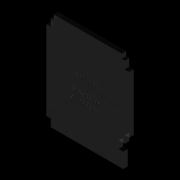
# Autodesk Inventor part: SideFaceBottomNM
Saved by Autodesk Inventor 2019 (Build 230136000, 136)
## iProperties
Created: 2019-05-08
Part Number: SideFaceBottomNM
Material: Acrylic, Clear
Document SubType Name: Modeling
Designer: super pig
Density: 1.19 g/cm^3
Appearance: Transparent - Black
Mass: 11.9621 g
Surface Area: 75.9473 cm^2
Volume: 10.0522 cm^3
Name: Bottom Face Cover
Author: super pig
Autodesk Inventor part; units mm, degrees
note: some values were not read from the file. Chosen so that the rebuilt part matches the saved one: direction of "Emboss1"; direction of "Emboss2".
ref_plane "YZ Plane" through (0, 0, 0) normal (1, 0, 0) x (0, 1, 0)
ref_plane "XZ Plane" through (0, 0, 0) normal (0, 1, 0) x (-1, 0, 0)
ref_plane "XY Plane" through (0, 0, 0) normal (0, 0, 1) x (1, 0, 0)
sketch "Sketch1" plane through (0, 0, 0) normal (0, 0, 1) x (1, 0, 0)
  line L0 (45, -52.75) -> (48, -52.75) projected
  line L1 (45, -52.75) -> (45, -62.75) projected
  line L2 (45, -62.75) -> (48, -62.75) projected
  line L3 (48, -52.75) -> (48, -62.75) projected
  line L4 (45, -47.75) -> (45, -52.75) projected
  line L5 (45, -52.75) -> (48, -52.75) projected
  line L6 (48, -47.75) -> (48, -52.75) projected
  line L7 (45, -47.75) -> (48, -47.75) projected
  line L8 (49, -42.75) -> (49, -47.75) projected
  line L9 (52, -42.75) -> (52, -47.75) projected
  line L10 (49, -42.75) -> (52, -42.75) projected
  line L11 (49, -5) -> (52, -5) projected
  line L12 (49, -5) -> (49, -42.75) projected
  line L13 (49, -42.75) -> (52, -42.75) projected
  line L14 (52, -5) -> (52, -42.75) projected
  line L15 (49, 0) -> (49, -5) projected
  line L16 (49, -5) -> (52, -5) projected
  line L17 (52, 0) -> (52, -5) projected
  line L18 (49, 0) -> (52, 0) projected
  line L19 (2, 3) -> (47, 3)
  line L20 (2, 0) -> (47, 0)
  line L21 (0, -5) -> (0, 0) projected
  line L22 (0, 0) -> (-3, 0) projected
  line L23 (-3, -5) -> (-3, 0) projected
  line L24 (0, -5) -> (-3, -5) projected
  line L25 (0, -57.75) -> (-3, -57.75) projected
  line L26 (0, -57.75) -> (0, -5) projected
  line L27 (-3, -57.75) -> (-3, -5) projected
  line L28 (0, -62.75) -> (0, -57.75) projected
  line L29 (0, -57.75) -> (-3, -57.75) projected
  line L30 (-3, -62.75) -> (-3, -57.75) projected
  line L31 (0, -62.75) -> (-3, -62.75) projected
  line L32 (48, -47.75) -> (49, -47.75)
  line L33 (45, -62.75) -> (0, -62.75)
  line L34 (49, -47.75) -> (52, -47.75) projected
  line L35 (0, -5) -> (-3, -5) projected
  line L36 (47, 3) -> (52, 3) projected
  line L37 (47, 0) -> (47, 3) projected
  line L38 (47, 0) -> (52, 0) projected
  line L39 (52, 0) -> (52, 3) projected
  line L40 (-3, 0) -> (2, 0) projected
  line L41 (2, 0) -> (2, 3) projected
  line L42 (-3, 3) -> (2, 3) projected
  line L43 (-3, 0) -> (-3, 3) projected
  constraints: 8 end point, 1 collinear, 1 horizontal
extrude "Extrusion1" add sketch "Sketch1" along normal blind 3 contours L0 L3 L2 L1 | L1 L33 L28 L26 L21 L40 L20 L38 L15 L12 L8 L32 L7 L4 | L25 L27 L24 L26 | L12 L11 L14 L10 | L41 L19 L37 L20
sketch "Sketch2" plane through (0, 0, 3) normal (0, 0, 1) x (1, 0, 0)
  circle A0 centre (38, -35.75) radius 4
  circle A1 centre (38, -23.75) radius 4
  line L0 (49, -47.75) -> (49, -42.75) projected
  line L1 (49, -42.75) -> (52, -42.75) projected
  point P0 (0, 0)
  point P1 (49, -5)
  dimension "d3" = 8
  dimension "d4" = 12
  dimension "d5" = 7
  dimension "d13" = 11
  constraints: 2 centre point, 1 equal radius, 1 vertical alignment
  measures "d3" diameter of A0
  measures "d4" distance of A0.centre A1.centre
  measures "d5" distance from line of L1 A0.centre
  measures "d13" distance from line of A0.centre L0
extrude "Extrusion2" cut sketch "Sketch2" against normal through all
sketch "Sketch3" plane through (0, 0, 3) normal (0, 0, 1) x (1, 0, 0)
  line L0 (45, -62.25) -> (0, -62.25) construction
  line L1 (0, -62.25) -> (0, -49.7711) construction
  line L2 (0, -49.7711) -> (45, -49.7711) construction
  line L3 (45, -49.7711) -> (45, -62.25) construction
  line L4 (45, -52.75) -> (45, -47.75) construction
  line L5 (0, -57.75) -> (0, -62.75) construction
  line L6 (0, -62.75) -> (48, -62.75) construction
  line L7 (42.4636, -61.6943) -> (42.9177, -61.6943)
  line L8 (42.9177, -61.6943) -> (42.9177, -60.9405)
  line L9 (42.9177, -60.9405) -> (43.1386, -60.9405)
  line L10 (43.1386, -60.9405) -> (43.1386, -61.6943)
  line L11 (43.1386, -61.6943) -> (43.5926, -61.6943)
  line L12 (43.5926, -61.6943) -> (43.5926, -61.7539)
  line L13 (43.5926, -61.7539) -> (43.0702, -62.3359)
  line L14 (43.0702, -62.3359) -> (42.9983, -62.3359)
  line L15 (42.9983, -62.3359) -> (42.4636, -61.7521)
  line L16 (42.4636, -61.7521) -> (42.4636, -61.6943)
  line L17 (38.7379, -59.294) -> (39.6954, -59.294)
  line L18 (39.6954, -59.294) -> (39.6954, -59.541)
  line L19 (39.6954, -59.541) -> (39.3488, -59.541)
  line L20 (39.3488, -59.541) -> (39.3488, -61.3891)
  line L21 (39.3488, -61.3891) -> (39.6954, -61.3891)
  line L22 (39.6954, -61.3891) -> (39.6954, -61.638)
  line L23 (39.6954, -61.638) -> (38.7379, -61.638)
  line L24 (38.7379, -61.638) -> (38.7379, -61.3891)
  line L25 (38.7379, -61.3891) -> (39.0845, -61.3891)
  line L26 (39.0845, -61.3891) -> (39.0845, -59.541)
  line L27 (39.0845, -59.541) -> (38.7379, -59.541)
  line L28 (38.7379, -59.541) -> (38.7379, -59.294)
  line L29 (36.48, -59.315) -> (36.6983, -59.315)
  line L30 (36.6983, -59.315) -> (37.9661, -61.1746)
  line L31 (37.9661, -61.1746) -> (37.9661, -59.315)
  line L32 (37.9661, -59.315) -> (38.2304, -59.315)
  line L33 (38.2304, -59.315) -> (38.2304, -61.6112)
  line L34 (38.2304, -61.6112) -> (38.0121, -61.617)
  line L35 (38.0121, -61.617) -> (36.7443, -59.7574)
  line L36 (36.7443, -59.7574) -> (36.7443, -61.615)
  line L37 (36.7443, -61.615) -> (36.48, -61.615)
  line L38 (36.48, -61.615) -> (36.48, -59.315)
  line L39 (34.2068, -59.7651) -> (34.699, -59.294)
  line L40 (34.699, -59.294) -> (35.5474, -59.294)
  line L41 (35.5474, -59.294) -> (36.0223, -59.7498)
  line L42 (36.0223, -59.7498) -> (35.848, -59.9145)
  line L43 (35.848, -59.9145) -> (35.442, -59.541)
  line L44 (35.442, -59.541) -> (34.8043, -59.541)
  line L45 (34.8043, -59.541) -> (34.5515, -59.7651)
  line L46 (34.5515, -59.7651) -> (36.0376, -61.1631)
  line L47 (36.0376, -61.1631) -> (35.5474, -61.638)
  line L48 (35.5474, -61.638) -> (34.699, -61.638)
  line L49 (34.699, -61.638) -> (34.2241, -61.1803)
  line L50 (34.2241, -61.1803) -> (34.3983, -61.0156)
  line L51 (34.3983, -61.0156) -> (34.8062, -61.3891)
  line L52 (34.8062, -61.3891) -> (35.442, -61.3891)
  line L53 (35.442, -61.3891) -> (35.6929, -61.1631)
  line L54 (35.6929, -61.1631) -> (34.2068, -59.7651)
  line L55 (32.039, -59.294) -> (33.7644, -59.294)
  line L56 (33.7644, -59.294) -> (33.7644, -61.638)
  line L57 (33.7644, -61.638) -> (32.039, -61.638)
  line L58 (32.039, -61.638) -> (32.039, -61.3891)
  line L59 (32.039, -61.3891) -> (33.5002, -61.3891)
  line L60 (33.5002, -61.3891) -> (33.5002, -60.5905)
  line L61 (33.5002, -60.5905) -> (32.782, -60.5905)
  line L62 (32.782, -60.5905) -> (32.782, -60.3396)
  line L63 (32.782, -60.3396) -> (33.5002, -60.3396)
  line L64 (33.5002, -60.3396) -> (33.5002, -59.541)
  line L65 (33.5002, -59.541) -> (32.039, -59.541)
  line L66 (32.039, -59.541) -> (32.039, -59.294)
  line L67 (29.7811, -60.7648) -> (30.2311, -60.3396)
  line L68 (30.2311, -60.3396) -> (30.754, -60.3396)
  line L69 (30.754, -60.3396) -> (29.7562, -59.4357)
  line L70 (29.7562, -59.4357) -> (29.9324, -59.271)
  line L71 (29.9324, -59.271) -> (31.0814, -60.3396)
  line L72 (31.0814, -60.3396) -> (31.2672, -60.3396)
  line L73 (31.2672, -60.3396) -> (31.2672, -59.315)
  line L74 (31.2672, -59.315) -> (31.5315, -59.315)
  line L75 (31.5315, -59.315) -> (31.5315, -61.638)
  line L76 (31.5315, -61.638) -> (30.2311, -61.638)
  line L77 (30.2311, -61.638) -> (29.7811, -61.2148)
  line L78 (29.7811, -61.2148) -> (29.7811, -60.7648)
  line L79 (30.0454, -60.8663) -> (30.0454, -61.1114)
  line L80 (30.0454, -61.1114) -> (30.3403, -61.3891)
  line L81 (30.3403, -61.3891) -> (31.2672, -61.3891)
  line L82 (31.2672, -61.3891) -> (31.2672, -60.5905)
  line L83 (31.2672, -60.5905) -> (30.3384, -60.5905)
  line L84 (30.3384, -60.5905) -> (30.0454, -60.8663)
  line L85 (27.573, -61.3891) -> (28.2912, -61.3891)
  line L86 (28.2912, -61.3891) -> (28.2912, -59.315)
  line L87 (28.2912, -59.315) -> (28.5555, -59.315)
  line L88 (28.5555, -59.315) -> (28.5555, -61.3891)
  line L89 (28.5555, -61.3891) -> (29.2736, -61.3891)
  line L90 (29.2736, -61.3891) -> (29.2736, -61.638)
  line L91 (29.2736, -61.638) -> (27.573, -61.638)
  line L92 (27.573, -61.638) -> (27.573, -61.3891)
  line L93 (23.1071, -59.294) -> (24.8326, -59.294)
  line L94 (24.8326, -59.294) -> (24.8326, -61.615)
  line L95 (24.8326, -61.615) -> (24.5683, -61.615)
  line L96 (24.5683, -61.615) -> (24.5683, -59.541)
  line L97 (24.5683, -59.541) -> (23.1071, -59.541)
  line L98 (23.1071, -59.541) -> (23.1071, -59.294)
  line L99 (20.8492, -59.315) -> (21.1135, -59.315)
  line L100 (21.1135, -59.315) -> (21.1135, -59.9911)
  line L101 (21.1135, -59.9911) -> (22.3353, -59.9911)
  line L102 (22.3353, -59.9911) -> (22.3353, -59.315)
  line L103 (22.3353, -59.315) -> (22.5996, -59.315)
  line L104 (22.5996, -59.315) -> (22.5996, -60.1462)
  line L105 (22.5996, -60.1462) -> (21.8201, -61.615)
  line L106 (21.8201, -61.615) -> (21.6286, -61.615)
  line L107 (21.6286, -61.615) -> (20.8492, -60.1462)
  line L108 (20.8492, -60.1462) -> (20.8492, -59.315)
  line L109 (21.1748, -60.2419) -> (21.7244, -61.2703)
  line L110 (21.7244, -61.2703) -> (22.2721, -60.2419)
  line L111 (22.2721, -60.2419) -> (21.1748, -60.2419)
  line L112 (18.5913, -59.7498) -> (19.0663, -59.294)
  line L113 (19.0663, -59.294) -> (19.9166, -59.294)
  line L114 (19.9166, -59.294) -> (20.3666, -59.7134)
  line L115 (20.3666, -59.7134) -> (20.3666, -61.2167)
  line L116 (20.3666, -61.2167) -> (19.9166, -61.638)
  line L117 (19.9166, -61.638) -> (19.0663, -61.638)
  line L118 (19.0663, -61.638) -> (18.5913, -61.1803)
  line L119 (18.5913, -61.1803) -> (18.7675, -61.0156)
  line L120 (18.7675, -61.0156) -> (19.1754, -61.3891)
  line L121 (19.1754, -61.3891) -> (19.8093, -61.3891)
  line L122 (19.8093, -61.3891) -> (20.1023, -61.1114)
  line L123 (20.1023, -61.1114) -> (20.1023, -59.8168)
  line L124 (20.1023, -59.8168) -> (19.8112, -59.541)
  line L125 (19.8112, -59.541) -> (19.1735, -59.541)
  line L126 (19.1735, -59.541) -> (18.7675, -59.9145)
  line L127 (18.7675, -59.9145) -> (18.5913, -59.7498)
  line L128 (16.4082, -59.294) -> (18.1336, -59.294)
  line L129 (18.1336, -59.294) -> (18.1336, -61.638)
  line L130 (18.1336, -61.638) -> (16.4082, -61.638)
  line L131 (16.4082, -61.638) -> (16.4082, -61.3891)
  line L132 (16.4082, -61.3891) -> (17.8694, -61.3891)
  line L133 (17.8694, -61.3891) -> (17.8694, -60.5905)
  line L134 (17.8694, -60.5905) -> (17.1512, -60.5905)
  line L135 (17.1512, -60.5905) -> (17.1512, -60.3396)
  line L136 (17.1512, -60.3396) -> (17.8694, -60.3396)
  line L137 (17.8694, -60.3396) -> (17.8694, -59.541)
  line L138 (17.8694, -59.541) -> (16.4082, -59.541)
  line L139 (16.4082, -59.541) -> (16.4082, -59.294)
  line L140 (11.9173, -59.315) -> (12.1816, -59.315)
  line L141 (12.1816, -59.315) -> (12.1816, -60.3396)
  line L142 (12.1816, -60.3396) -> (13.4034, -60.3396)
  line L143 (13.4034, -60.3396) -> (13.4034, -59.315)
  line L144 (13.4034, -59.315) -> (13.6677, -59.315)
  line L145 (13.6677, -59.315) -> (13.6677, -61.615)
  line L146 (13.6677, -61.615) -> (13.4034, -61.615)
  line L147 (13.4034, -61.615) -> (13.4034, -60.5905)
  line L148 (13.4034, -60.5905) -> (12.1816, -60.5905)
  line L149 (12.1816, -60.5905) -> (12.1816, -61.615)
  line L150 (12.1816, -61.615) -> (11.9173, -61.615)
  line L151 (11.9173, -61.615) -> (11.9173, -59.315)
  line L152 (9.7092, -59.294) -> (11.4347, -59.294)
  line L153 (11.4347, -59.294) -> (11.4347, -61.638)
  line L154 (11.4347, -61.638) -> (9.7092, -61.638)
  line L155 (9.7092, -61.638) -> (9.7092, -61.3891)
  line L156 (9.7092, -61.3891) -> (11.1704, -61.3891)
  line L157 (11.1704, -61.3891) -> (11.1704, -60.5905)
  line L158 (11.1704, -60.5905) -> (10.4523, -60.5905)
  line L159 (10.4523, -60.5905) -> (10.4523, -60.3396)
  line L160 (10.4523, -60.3396) -> (11.1704, -60.3396)
  line L161 (11.1704, -60.3396) -> (11.1704, -59.541)
  line L162 (11.1704, -59.541) -> (9.7092, -59.541)
  line L163 (9.7092, -59.541) -> (9.7092, -59.294)
  line L164 (7.4514, -60.7648) -> (7.9014, -60.3396)
  line L165 (7.9014, -60.3396) -> (8.4242, -60.3396)
  line L166 (8.4242, -60.3396) -> (7.4265, -59.4357)
  line L167 (7.4265, -59.4357) -> (7.6027, -59.271)
  line L168 (7.6027, -59.271) -> (8.7517, -60.3396)
  line L169 (8.7517, -60.3396) -> (8.9375, -60.3396)
  line L170 (8.9375, -60.3396) -> (8.9375, -59.315)
  line L171 (8.9375, -59.315) -> (9.2017, -59.315)
  line L172 (9.2017, -59.315) -> (9.2017, -61.638)
  line L173 (9.2017, -61.638) -> (7.9014, -61.638)
  line L174 (7.9014, -61.638) -> (7.4514, -61.2148)
  line L175 (7.4514, -61.2148) -> (7.4514, -60.7648)
  line L176 (7.7157, -60.8663) -> (7.7157, -61.1114)
  line L177 (7.7157, -61.1114) -> (8.0106, -61.3891)
  line L178 (8.0106, -61.3891) -> (8.9375, -61.3891)
  line L179 (8.9375, -61.3891) -> (8.9375, -60.5905)
  line L180 (8.9375, -60.5905) -> (8.0087, -60.5905)
  line L181 (8.0087, -60.5905) -> (7.7157, -60.8663)
  line L182 (5.2433, -59.294) -> (6.9688, -59.294)
  line L183 (6.9688, -59.294) -> (6.9688, -61.638)
  line L184 (6.9688, -61.638) -> (5.2433, -61.638)
  line L185 (5.2433, -61.638) -> (5.2433, -61.3891)
  line L186 (5.2433, -61.3891) -> (6.7045, -61.3891)
  line L187 (6.7045, -61.3891) -> (6.7045, -60.5905)
  line L188 (6.7045, -60.5905) -> (5.9863, -60.5905)
  line L189 (5.9863, -60.5905) -> (5.9863, -60.3396)
  line L190 (5.9863, -60.3396) -> (6.7045, -60.3396)
  line L191 (6.7045, -60.3396) -> (6.7045, -59.541)
  line L192 (6.7045, -59.541) -> (5.2433, -59.541)
  line L193 (5.2433, -59.541) -> (5.2433, -59.294)
  line L194 (1.4056, -61.6943) -> (1.8597, -61.6943)
  line L195 (1.8597, -61.6943) -> (1.8597, -60.9405)
  line L196 (1.8597, -60.9405) -> (2.0806, -60.9405)
  line L197 (2.0806, -60.9405) -> (2.0806, -61.6943)
  line L198 (2.0806, -61.6943) -> (2.5346, -61.6943)
  line L199 (2.5346, -61.6943) -> (2.5346, -61.7539)
  line L200 (2.5346, -61.7539) -> (2.0122, -62.3359)
  line L201 (2.0122, -62.3359) -> (1.9403, -62.3359)
  line L202 (1.9403, -62.3359) -> (1.4056, -61.7521)
  line L203 (1.4056, -61.7521) -> (1.4056, -61.6943)
  point P0 (0, 0)
  point P1 (22.5, -62.25)
  point P2 (45, -62.75)
  point P3 (0, -52.75)
  point P4 (0, -5)
  dimension "d8" = 0.5
  constraints: 2 vertical alignment, 1 horizontal, 1 midpoint, 2 other
  measures "d8" distance between parallel lines of L6 L0
emboss "Emboss1" sketch "Sketch3" operation cut depth 0.1 direction (0, 0, -1)
sketch "Sketch4" plane through (0, 0, 3) normal (0, 0, 1) x (1, 0, 0)
  line L0 (34, -41.7398) -> (9.9219, -41.7398) construction
  line L1 (9.9219, -41.7398) -> (9.9219, -29.7602) construction
  line L2 (9.9219, -29.7602) -> (34, -29.7602) construction
  line L3 (34, -29.7602) -> (34, -41.7398) construction
  circle A0 centre (38, -35.75) radius 4 construction
  line L4 (34, -27.7943) -> (9.9219, -27.7943) construction
  line L5 (9.9219, -27.7943) -> (9.9219, -19.7057) construction
  line L6 (9.9219, -19.7057) -> (34, -19.7057) construction
  line L7 (34, -19.7057) -> (34, -27.7943) construction
  circle A1 centre (38, -23.75) radius 4 construction
  line L8 (29.1157, -38.4984) -> (29.5594, -38.0797)
  line L9 (29.5594, -38.0797) -> (30.1171, -38.0797)
  line L10 (30.1171, -38.0797) -> (29.0925, -37.1208)
  line L11 (29.0925, -37.1208) -> (29.2391, -36.9838)
  line L12 (29.2391, -36.9838) -> (30.4084, -38.0797)
  line L13 (30.4084, -38.0797) -> (30.6438, -38.0797)
  line L14 (30.6438, -38.0797) -> (30.6438, -37.0281)
  line L15 (30.6438, -37.0281) -> (30.8503, -37.0281)
  line L16 (30.8503, -37.0281) -> (30.8503, -39.3513)
  line L17 (30.8503, -39.3513) -> (29.5594, -39.3513)
  line L18 (29.5594, -39.3513) -> (29.1157, -38.9364)
  line L19 (29.1157, -38.9364) -> (29.1157, -38.4984)
  line L20 (29.324, -38.5775) -> (29.324, -38.8554)
  line L21 (29.324, -38.8554) -> (29.6443, -39.1583)
  line L22 (29.6443, -39.1583) -> (30.6438, -39.1583)
  line L23 (30.6438, -39.1583) -> (30.6438, -38.2746)
  line L24 (30.6438, -38.2746) -> (29.6443, -38.2746)
  line L25 (29.6443, -38.2746) -> (29.324, -38.5775)
  line L26 (26.8504, -37.0069) -> (28.558, -37.0069)
  line L27 (28.558, -37.0069) -> (28.558, -39.3513)
  line L28 (28.558, -39.3513) -> (26.8504, -39.3513)
  line L29 (26.8504, -39.3513) -> (26.8504, -39.1583)
  line L30 (26.8504, -39.1583) -> (28.3516, -39.1583)
  line L31 (28.3516, -39.1583) -> (28.3516, -38.2746)
  line L32 (28.3516, -38.2746) -> (27.6145, -38.2746)
  line L33 (27.6145, -38.2746) -> (27.6145, -38.0797)
  line L34 (27.6145, -38.0797) -> (28.3516, -38.0797)
  line L35 (28.3516, -38.0797) -> (28.3516, -37.1979)
  line L36 (28.3516, -37.1979) -> (26.8504, -37.1979)
  line L37 (26.8504, -37.1979) -> (26.8504, -37.0069)
  line L38 (24.5581, -37.0069) -> (26.2657, -37.0069)
  line L39 (26.2657, -37.0069) -> (26.2657, -39.3281)
  line L40 (26.2657, -39.3281) -> (26.0593, -39.3281)
  line L41 (26.0593, -39.3281) -> (26.0593, -37.1979)
  line L42 (26.0593, -37.1979) -> (24.5581, -37.1979)
  line L43 (24.5581, -37.1979) -> (24.5581, -37.0069)
  line L44 (22.2658, -37.0069) -> (23.9735, -37.0069)
  line L45 (23.9735, -37.0069) -> (23.9735, -39.3513)
  line L46 (23.9735, -39.3513) -> (22.2658, -39.3513)
  line L47 (22.2658, -39.3513) -> (22.2658, -39.1583)
  line L48 (22.2658, -39.1583) -> (23.767, -39.1583)
  line L49 (23.767, -39.1583) -> (23.767, -38.2746)
  line L50 (23.767, -38.2746) -> (23.0299, -38.2746)
  line L51 (23.0299, -38.2746) -> (23.0299, -38.0797)
  line L52 (23.0299, -38.0797) -> (23.767, -38.0797)
  line L53 (23.767, -38.0797) -> (23.767, -37.1979)
  line L54 (23.767, -37.1979) -> (22.2658, -37.1979)
  line L55 (22.2658, -37.1979) -> (22.2658, -37.0069)
  line L56 (19.9465, -37.0281) -> (20.1549, -37.0281)
  line L57 (20.1549, -37.0281) -> (20.1549, -37.7228)
  line L58 (20.1549, -37.7228) -> (21.4747, -37.7228)
  line L59 (21.4747, -37.7228) -> (21.4747, -37.0281)
  line L60 (21.4747, -37.0281) -> (21.6812, -37.0281)
  line L61 (21.6812, -37.0281) -> (21.6812, -37.8424)
  line L62 (21.6812, -37.8424) -> (20.892, -39.3281)
  line L63 (20.892, -39.3281) -> (20.7376, -39.3281)
  line L64 (20.7376, -39.3281) -> (19.9465, -37.8424)
  line L65 (19.9465, -37.8424) -> (19.9465, -37.0281)
  line L66 (20.2186, -37.9176) -> (20.8148, -39.0368)
  line L67 (20.8148, -39.0368) -> (21.411, -37.9176)
  line L68 (21.411, -37.9176) -> (20.2186, -37.9176)
  line L69 (17.6157, -37.4584) -> (18.1, -37.0069)
  line L70 (18.1, -37.0069) -> (18.947, -37.0069)
  line L71 (18.947, -37.0069) -> (19.4159, -37.443)
  line L72 (19.4159, -37.443) -> (19.2673, -37.5819)
  line L73 (19.2673, -37.5819) -> (18.8641, -37.1979)
  line L74 (18.8641, -37.1979) -> (18.1829, -37.1979)
  line L75 (18.1829, -37.1979) -> (17.9032, -37.4584)
  line L76 (17.9032, -37.4584) -> (19.4313, -38.8959)
  line L77 (19.4313, -38.8959) -> (18.947, -39.3513)
  line L78 (18.947, -39.3513) -> (18.1, -39.3513)
  line L79 (18.1, -39.3513) -> (17.6311, -38.9133)
  line L80 (17.6311, -38.9133) -> (17.7777, -38.7744)
  line L81 (17.7777, -38.7744) -> (18.1829, -39.1583)
  line L82 (18.1829, -39.1583) -> (18.8641, -39.1583)
  line L83 (18.8641, -39.1583) -> (19.1419, -38.8959)
  line L84 (19.1419, -38.8959) -> (17.6157, -37.4584)
  line L85 (15.389, -37.0069) -> (17.0966, -37.0069)
  line L86 (17.0966, -37.0069) -> (17.0966, -39.3513)
  line L87 (17.0966, -39.3513) -> (15.389, -39.3513)
  line L88 (15.389, -39.3513) -> (15.389, -39.1583)
  line L89 (15.389, -39.1583) -> (16.8902, -39.1583)
  line L90 (16.8902, -39.1583) -> (16.8902, -38.2746)
  line L91 (16.8902, -38.2746) -> (16.1531, -38.2746)
  line L92 (16.1531, -38.2746) -> (16.1531, -38.0797)
  line L93 (16.1531, -38.0797) -> (16.8902, -38.0797)
  line L94 (16.8902, -38.0797) -> (16.8902, -37.1979)
  line L95 (16.8902, -37.1979) -> (15.389, -37.1979)
  line L96 (15.389, -37.1979) -> (15.389, -37.0069)
  line L97 (13.0388, -39.2683) -> (14.6558, -36.9953)
  line L98 (14.6558, -36.9953) -> (14.8333, -37.0899)
  line L99 (14.8333, -37.0899) -> (13.2221, -39.3629)
  line L100 (13.2221, -39.3629) -> (13.0388, -39.2683)
  line L101 (29.8797, -32.1584) -> (30.0881, -32.1584)
  line L102 (30.0881, -32.1584) -> (30.0881, -32.853)
  line L103 (30.0881, -32.853) -> (31.4079, -32.853)
  line L104 (31.4079, -32.853) -> (31.4079, -32.1584)
  line L105 (31.4079, -32.1584) -> (31.6144, -32.1584)
  line L106 (31.6144, -32.1584) -> (31.6144, -32.9726)
  line L107 (31.6144, -32.9726) -> (30.8252, -34.4584)
  line L108 (30.8252, -34.4584) -> (30.6709, -34.4584)
  line L109 (30.6709, -34.4584) -> (29.8797, -32.9726)
  line L110 (29.8797, -32.9726) -> (29.8797, -32.1584)
  line L111 (30.1518, -33.0479) -> (30.748, -34.167)
  line L112 (30.748, -34.167) -> (31.3443, -33.0479)
  line L113 (31.3443, -33.0479) -> (30.1518, -33.0479)
  line L114 (27.5643, -32.5732) -> (28.0313, -32.1371)
  line L115 (28.0313, -32.1371) -> (28.8803, -32.1371)
  line L116 (28.8803, -32.1371) -> (29.3221, -32.5501)
  line L117 (29.3221, -32.5501) -> (29.3221, -34.0667)
  line L118 (29.3221, -34.0667) -> (28.8803, -34.4815)
  line L119 (28.8803, -34.4815) -> (28.0313, -34.4815)
  line L120 (28.0313, -34.4815) -> (27.5643, -34.0435)
  line L121 (27.5643, -34.0435) -> (27.711, -33.9046)
  line L122 (27.711, -33.9046) -> (28.1162, -34.2886)
  line L123 (28.1162, -34.2886) -> (28.7954, -34.2886)
  line L124 (28.7954, -34.2886) -> (29.1157, -33.9856)
  line L125 (29.1157, -33.9856) -> (29.1157, -32.6292)
  line L126 (29.1157, -32.6292) -> (28.7954, -32.3282)
  line L127 (28.7954, -32.3282) -> (28.1162, -32.3282)
  line L128 (28.1162, -32.3282) -> (27.711, -32.7121)
  line L129 (27.711, -32.7121) -> (27.5643, -32.5732)
  line L130 (25.3222, -34.2886) -> (26.0612, -34.2886)
  line L131 (26.0612, -34.2886) -> (26.0612, -32.1584)
  line L132 (26.0612, -32.1584) -> (26.2677, -32.1584)
  line L133 (26.2677, -32.1584) -> (26.2677, -34.2886)
  line L134 (26.2677, -34.2886) -> (27.0047, -34.2886)
  line L135 (27.0047, -34.2886) -> (27.0047, -34.4815)
  line L136 (27.0047, -34.4815) -> (25.3222, -34.4815)
  line L137 (25.3222, -34.4815) -> (25.3222, -34.2886)
  line L138 (23.794, -32.1371) -> (24.7125, -32.1371)
  line L139 (24.7125, -32.1371) -> (24.7125, -32.3282)
  line L140 (24.7125, -32.3282) -> (24.3555, -32.3282)
  line L141 (24.3555, -32.3282) -> (24.3555, -34.2886)
  line L142 (24.3555, -34.2886) -> (24.7125, -34.2886)
  line L143 (24.7125, -34.2886) -> (24.7125, -34.4815)
  line L144 (24.7125, -34.4815) -> (23.794, -34.4815)
  line L145 (23.794, -34.4815) -> (23.794, -34.2886)
  line L146 (23.794, -34.2886) -> (24.151, -34.2886)
  line L147 (24.151, -34.2886) -> (24.151, -32.3282)
  line L148 (24.151, -32.3282) -> (23.794, -32.3282)
  line L149 (23.794, -32.3282) -> (23.794, -32.1371)
  line L150 (20.6913, -34.4043) -> (21.8857, -32.1584)
  line L151 (21.8857, -32.1584) -> (22.0381, -32.1584)
  line L152 (22.0381, -32.1584) -> (23.2306, -34.4043)
  line L153 (23.2306, -34.4043) -> (23.0531, -34.5008)
  line L154 (23.0531, -34.5008) -> (21.9629, -32.4478)
  line L155 (21.9629, -32.4478) -> (20.8727, -34.4989)
  line L156 (20.8727, -34.4989) -> (20.6913, -34.4043)
  line L157 (19.2094, -32.1371) -> (20.1279, -32.1371)
  line L158 (20.1279, -32.1371) -> (20.1279, -32.3282)
  line L159 (20.1279, -32.3282) -> (19.7709, -32.3282)
  line L160 (19.7709, -32.3282) -> (19.7709, -34.2886)
  line L161 (19.7709, -34.2886) -> (20.1279, -34.2886)
  line L162 (20.1279, -34.2886) -> (20.1279, -34.4815)
  line L163 (20.1279, -34.4815) -> (19.2094, -34.4815)
  line L164 (19.2094, -34.4815) -> (19.2094, -34.2886)
  line L165 (19.2094, -34.2886) -> (19.5664, -34.2886)
  line L166 (19.5664, -34.2886) -> (19.5664, -32.3282)
  line L167 (19.5664, -32.3282) -> (19.2094, -32.3282)
  line L168 (19.2094, -32.3282) -> (19.2094, -32.1371)
  line L169 (16.8902, -32.1584) -> (17.0985, -32.1584)
  line L170 (17.0985, -32.1584) -> (17.0985, -32.853)
  line L171 (17.0985, -32.853) -> (18.4183, -32.853)
  line L172 (18.4183, -32.853) -> (18.4183, -32.1584)
  line L173 (18.4183, -32.1584) -> (18.6248, -32.1584)
  line L174 (18.6248, -32.1584) -> (18.6248, -32.9726)
  line L175 (18.6248, -32.9726) -> (17.8356, -34.4584)
  line L176 (17.8356, -34.4584) -> (17.6813, -34.4584)
  line L177 (17.6813, -34.4584) -> (16.8902, -32.9726)
  line L178 (16.8902, -32.9726) -> (16.8902, -32.1584)
  line L179 (17.1622, -33.0479) -> (17.7584, -34.167)
  line L180 (17.7584, -34.167) -> (18.3547, -33.0479)
  line L181 (18.3547, -33.0479) -> (17.1622, -33.0479)
  line L182 (14.6249, -34.2886) -> (15.3639, -34.2886)
  line L183 (15.3639, -34.2886) -> (15.3639, -32.1584)
  line L184 (15.3639, -32.1584) -> (15.5704, -32.1584)
  line L185 (15.5704, -32.1584) -> (15.5704, -34.2886)
  line L186 (15.5704, -34.2886) -> (16.3074, -34.2886)
  line L187 (16.3074, -34.2886) -> (16.3074, -34.4815)
  line L188 (16.3074, -34.4815) -> (14.6249, -34.4815)
  line L189 (14.6249, -34.4815) -> (14.6249, -34.2886)
  line L190 (12.3326, -32.1371) -> (14.0402, -32.1371)
  line L191 (14.0402, -32.1371) -> (14.0402, -34.4815)
  line L192 (14.0402, -34.4815) -> (12.3326, -34.4815)
  line L193 (12.3326, -34.4815) -> (12.3326, -34.2886)
  line L194 (12.3326, -34.2886) -> (13.8338, -34.2886)
  line L195 (13.8338, -34.2886) -> (13.8338, -33.4048)
  line L196 (13.8338, -33.4048) -> (13.0967, -33.4048)
  line L197 (13.0967, -33.4048) -> (13.0967, -33.21)
  line L198 (13.0967, -33.21) -> (13.8338, -33.21)
  line L199 (13.8338, -33.21) -> (13.8338, -32.3282)
  line L200 (13.8338, -32.3282) -> (12.3326, -32.3282)
  line L201 (12.3326, -32.3282) -> (12.3326, -32.1371)
  line L202 (29.1157, -24.0809) -> (29.5594, -23.6622)
  line L203 (29.5594, -23.6622) -> (30.6438, -23.6622)
  line L204 (30.6438, -23.6622) -> (30.6438, -22.6106)
  line L205 (30.6438, -22.6106) -> (30.8503, -22.6106)
  line L206 (30.8503, -22.6106) -> (30.8503, -24.9338)
  line L207 (30.8503, -24.9338) -> (29.5594, -24.9338)
  line L208 (29.5594, -24.9338) -> (29.1157, -24.5189)
  line L209 (29.1157, -24.5189) -> (29.1157, -24.0809)
  line L210 (29.324, -24.16) -> (29.324, -24.4379)
  line L211 (29.324, -24.4379) -> (29.6443, -24.7408)
  line L212 (29.6443, -24.7408) -> (30.6438, -24.7408)
  line L213 (30.6438, -24.7408) -> (30.6438, -23.8571)
  line L214 (30.6438, -23.8571) -> (29.6443, -23.8571)
  line L215 (29.6443, -23.8571) -> (29.324, -24.16)
  line L216 (26.8234, -24.0809) -> (27.2672, -23.6622)
  line L217 (27.2672, -23.6622) -> (27.8248, -23.6622)
  line L218 (27.8248, -23.6622) -> (26.8002, -22.7032)
  line L219 (26.8002, -22.7032) -> (26.9469, -22.5662)
  line L220 (26.9469, -22.5662) -> (28.1162, -23.6622)
  line L221 (28.1162, -23.6622) -> (28.3516, -23.6622)
  line L222 (28.3516, -23.6622) -> (28.3516, -22.6106)
  line L223 (28.3516, -22.6106) -> (28.558, -22.6106)
  line L224 (28.558, -22.6106) -> (28.558, -24.9338)
  line L225 (28.558, -24.9338) -> (27.2672, -24.9338)
  line L226 (27.2672, -24.9338) -> (26.8234, -24.5189)
  line L227 (26.8234, -24.5189) -> (26.8234, -24.0809)
  line L228 (27.0318, -24.16) -> (27.0318, -24.4379)
  line L229 (27.0318, -24.4379) -> (27.3521, -24.7408)
  line L230 (27.3521, -24.7408) -> (28.3516, -24.7408)
  line L231 (28.3516, -24.7408) -> (28.3516, -23.8571)
  line L232 (28.3516, -23.8571) -> (27.3521, -23.8571)
  line L233 (27.3521, -23.8571) -> (27.0318, -24.16)
  line L234 (24.5581, -22.5894) -> (26.2657, -22.5894)
  line L235 (26.2657, -22.5894) -> (26.2657, -24.9338)
  line L236 (26.2657, -24.9338) -> (24.5581, -24.9338)
  line L237 (24.5581, -24.9338) -> (24.5581, -24.7408)
  line L238 (24.5581, -24.7408) -> (26.0593, -24.7408)
  line L239 (26.0593, -24.7408) -> (26.0593, -23.8571)
  line L240 (26.0593, -23.8571) -> (25.3222, -23.8571)
  line L241 (25.3222, -23.8571) -> (25.3222, -23.6622)
  line L242 (25.3222, -23.6622) -> (26.0593, -23.6622)
  line L243 (26.0593, -23.6622) -> (26.0593, -22.7804)
  line L244 (26.0593, -22.7804) -> (24.5581, -22.7804)
  line L245 (24.5581, -22.7804) -> (24.5581, -22.5894)
  line L246 (22.2002, -23.0409) -> (22.6845, -22.5894)
  line L247 (22.6845, -22.5894) -> (23.5316, -22.5894)
  line L248 (23.5316, -22.5894) -> (24.0005, -23.0255)
  line L249 (24.0005, -23.0255) -> (23.8519, -23.1644)
  line L250 (23.8519, -23.1644) -> (23.4486, -22.7804)
  line L251 (23.4486, -22.7804) -> (22.7675, -22.7804)
  line L252 (22.7675, -22.7804) -> (22.4877, -23.0409)
  line L253 (22.4877, -23.0409) -> (24.0159, -24.4784)
  line L254 (24.0159, -24.4784) -> (23.5316, -24.9338)
  line L255 (23.5316, -24.9338) -> (22.6845, -24.9338)
  line L256 (22.6845, -24.9338) -> (22.2157, -24.4958)
  line L257 (22.2157, -24.4958) -> (22.3623, -24.3568)
  line L258 (22.3623, -24.3568) -> (22.7675, -24.7408)
  line L259 (22.7675, -24.7408) -> (23.4486, -24.7408)
  line L260 (23.4486, -24.7408) -> (23.7265, -24.4784)
  line L261 (23.7265, -24.4784) -> (22.2002, -23.0409)
  line L262 (19.9079, -23.0409) -> (20.3922, -22.5894)
  line L263 (20.3922, -22.5894) -> (21.2393, -22.5894)
  line L264 (21.2393, -22.5894) -> (21.7082, -23.0255)
  line L265 (21.7082, -23.0255) -> (21.5596, -23.1644)
  line L266 (21.5596, -23.1644) -> (21.1563, -22.7804)
  line L267 (21.1563, -22.7804) -> (20.4752, -22.7804)
  line L268 (20.4752, -22.7804) -> (20.1954, -23.0409)
  line L269 (20.1954, -23.0409) -> (21.7236, -24.4784)
  line L270 (21.7236, -24.4784) -> (21.2393, -24.9338)
  line L271 (21.2393, -24.9338) -> (20.3922, -24.9338)
  line L272 (20.3922, -24.9338) -> (19.9234, -24.4958)
  line L273 (19.9234, -24.4958) -> (20.07, -24.3568)
  line L274 (20.07, -24.3568) -> (20.4752, -24.7408)
  line L275 (20.4752, -24.7408) -> (21.1563, -24.7408)
  line L276 (21.1563, -24.7408) -> (21.4342, -24.4784)
  line L277 (21.4342, -24.4784) -> (19.9079, -23.0409)
  line L278 (17.6542, -23.0023) -> (18.098, -22.5894)
  line L279 (18.098, -22.5894) -> (18.947, -22.5894)
  line L280 (18.947, -22.5894) -> (19.3889, -23.0023)
  line L281 (19.3889, -23.0023) -> (19.3889, -24.9106)
  line L282 (19.3889, -24.9106) -> (19.1824, -24.9106)
  line L283 (19.1824, -24.9106) -> (19.1824, -23.0814)
  line L284 (19.1824, -23.0814) -> (18.8621, -22.7804)
  line L285 (18.8621, -22.7804) -> (18.1829, -22.7804)
  line L286 (18.1829, -22.7804) -> (17.8626, -23.0814)
  line L287 (17.8626, -23.0814) -> (17.8626, -24.9106)
  line L288 (17.8626, -24.9106) -> (17.6542, -24.9106)
  line L289 (17.6542, -24.9106) -> (17.6542, -23.0023)
  line L290 (15.362, -24.0809) -> (15.8058, -23.6622)
  line L291 (15.8058, -23.6622) -> (16.3634, -23.6622)
  line L292 (16.3634, -23.6622) -> (15.3388, -22.7032)
  line L293 (15.3388, -22.7032) -> (15.4855, -22.5662)
  line L294 (15.4855, -22.5662) -> (16.6547, -23.6622)
  line L295 (16.6547, -23.6622) -> (16.8902, -23.6622)
  line L296 (16.8902, -23.6622) -> (16.8902, -22.6106)
  line L297 (16.8902, -22.6106) -> (17.0966, -22.6106)
  line L298 (17.0966, -22.6106) -> (17.0966, -24.9338)
  line L299 (17.0966, -24.9338) -> (15.8058, -24.9338)
  line L300 (15.8058, -24.9338) -> (15.362, -24.5189)
  line L301 (15.362, -24.5189) -> (15.362, -24.0809)
  line L302 (15.5704, -24.16) -> (15.5704, -24.4379)
  line L303 (15.5704, -24.4379) -> (15.8907, -24.7408)
  line L304 (15.8907, -24.7408) -> (16.8902, -24.7408)
  line L305 (16.8902, -24.7408) -> (16.8902, -23.8571)
  line L306 (16.8902, -23.8571) -> (15.8907, -23.8571)
  line L307 (15.8907, -23.8571) -> (15.5704, -24.16)
  line L308 (13.0967, -22.5894) -> (14.8043, -22.5894)
  line L309 (14.8043, -22.5894) -> (14.8043, -24.9338)
  line L310 (14.8043, -24.9338) -> (13.0967, -24.9338)
  line L311 (13.0967, -24.9338) -> (13.0967, -24.7408)
  line L312 (13.0967, -24.7408) -> (14.5979, -24.7408)
  line L313 (14.5979, -24.7408) -> (14.5979, -23.8571)
  line L314 (14.5979, -23.8571) -> (13.8608, -23.8571)
  line L315 (13.8608, -23.8571) -> (13.8608, -23.6622)
  line L316 (13.8608, -23.6622) -> (14.5979, -23.6622)
  line L317 (14.5979, -23.6622) -> (14.5979, -22.7804)
  line L318 (14.5979, -22.7804) -> (13.0967, -22.7804)
  line L319 (13.0967, -22.7804) -> (13.0967, -22.5894)
  point P0 (0, 0)
  point P1 (34, -35.75)
  point P2 (34, -23.75)
  constraints: 4 horizontal alignment, 2 midpoint, 1 vertical alignment, 6 other
emboss "Emboss2" sketch "Sketch4" operation cut depth 0.25 direction (0, 0, -1)
body "Solid1"
